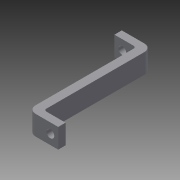
# Autodesk Inventor part: MotorBracket
Saved by Autodesk Inventor 2015 (Build 190159000, 159)
## iProperties
Created: 2017-03-10
Part Number: MotorBracket
Material: Generic
Document SubType Name: Modeling
Designer: 1esh9
Density: 1 g/cm^3
Appearance: Default
Author: 1esh9
Autodesk Inventor part; units mm, degrees
ref_plane "YZ Plane" through (0, 0, 0) normal (1, 0, 0) x (0, 1, 0)
ref_plane "XZ Plane" through (0, 0, 0) normal (0, 1, 0) x (-1, 0, 0)
ref_plane "XY Plane" through (0, 0, 0) normal (0, 0, 1) x (1, 0, 0)
sketch "Sketch1" plane through (0, 0, 0) normal (0, 0, 1) x (1, 0, 0)
  line L0 (0, 0) -> (3.4, 0)
  line L1 (3.4, 0) -> (3.4, 44)
  line L2 (3.4, 44) -> (0, 44)
  line L3 (0, 44) -> (0, 0)
  line L4 (3.4, 44) -> (-8.85, 44)
  line L5 (-8.85, 44) -> (-8.85, 47)
  line L6 (-8.85, 47) -> (3.4, 47)
  line L7 (3.4, 47) -> (3.4, 44)
  line L8 (3.4, 0) -> (12.25, 0)
  line L9 (12.25, 0) -> (12.25, 3)
  line L10 (12.25, 3) -> (3.4, 3)
  line L11 (3.4, 3) -> (3.4, 0)
  line L12 (-5.65, 47) -> (-5.65, 44) construction
  line L13 (-7.25, 47) -> (-7.25, 44) construction
  line L14 (-4.05, 44) -> (-4.05, 47) construction
  dimension "d0" = 44
  dimension "d1" = 3.4
  dimension "d3" = 5.65
  dimension "d4" = 3.2
  dimension "d5" = 1.6
  dimension "d6" = 1.6
  dimension "d7" = 3
  dimension "d8" = 3
  dimension "d9" = 12.25
  dimension "d10" = 12.25
  constraints: 30 end point, 6 parallel, 6 perpendicular, 6 point on line, 3 horizontal
  measures "d0" distance of L2.end L0.start
  measures "d1" distance of L1.end L2.end
  measures "d3" distance between parallel lines of L3 L12
  measures "d4" distance between parallel lines of L14 L13
  measures "d5" distance between parallel lines of L12 L13
  measures "d6" distance between parallel lines of L13 L5
  measures "d7" distance of L4.end L5.end
  measures "d8" distance of L8.end L9.end
  measures "d9" distance between parallel lines of L7 L5
  measures "d10" distance between parallel lines of L3 L9
extrude "Extrusion1" add sketch "Sketch1" along normal blind 8
sketch "Sketch2" plane through (-8.85, 47, 0) normal (0, 1, 0) x (1, 0, 0)
  line L0 (12.25, 0) -> (0, 0) projected
  line L1 (0, 0) -> (0, -8) projected
  line L2 (12.25, -8) -> (0, -8) projected
  line L3 (12.25, 0) -> (12.25, -8) projected
  line L4 (21.1, 0) -> (12.25, 0) projected
  line L5 (12.25, 0) -> (12.25, -8) projected
  line L6 (21.1, -8) -> (12.25, -8) projected
  line L7 (21.1, 0) -> (21.1, -8) projected
  circle A0 centre (3.2, -4) radius 1.6
  circle A1 centre (17.9, -4) radius 1.6
  point P0 (8.85, 0)
  dimension "d13" = 3.2
  dimension "d14" = 3.2
  dimension "d15" = 3.2
  dimension "d16" = 3.2
  constraints: 2 centre point
  measures "d13" diameter of A0
  measures "d14" diameter of A1
  measures "d15" distance from line of L1 A0.centre
  measures "d16" distance from line of L7 A1.centre
extrude "Extrusion2" cut sketch "Sketch2" against normal blind 51.5 contours A0 | A1
fillet "Fillet1" radius 3 2 edges at (3.4, 47, 4) (0, 0, 4)
fillet "Fillet2" radius 1 2 edges at (3.4, 3, 4) (0, 44, 4)
equation "\"d5\" = 0.5 * d4"
equation "\"d6\" = d5"
equation "\"d10\" = d9"
body "Solid1"
